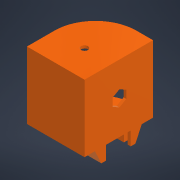
# Autodesk Inventor part: Base
Saved by Autodesk Inventor 2022 (Build 260153000, 153)
## iProperties
Created: 2021-06-04
Part Number: Base
Material: Generic
Document SubType Name: Modeling
Designer: saatvik123
Density: 1 g/cm^3
Appearance: Smooth - Light Orange
Author: saatvik123
## iProperties of the stored document Base_3DPrint.ipt
Created: 2021-06-05
Part Number: Base_3DPrint
Material: Generic
Document SubType Name: Modeling
Designer: sidsa
Density: 1 g/cm^3
Appearance: Default
Author: sidsa
Autodesk Inventor part; units mm, degrees
ref_plane "YZ Plane" through (0, 0, 0) normal (1, 0, 0) x (0, 1, 0)
ref_plane "XZ Plane" through (0, 0, 0) normal (0, 1, 0) x (-1, 0, 0)
ref_plane "XY Plane" through (0, 0, 0) normal (0, 0, 1) x (1, 0, 0)
sketch "Sketch1" plane through (0, 0, 0) normal (0, 0, 1) x (1, 0, 0)
  line L0 (-30.48, 28.575) -> (20.32, 28.575)
  line L1 (20.32, 28.575) -> (20.32, -28.575)
  line L2 (20.32, -28.575) -> (-30.48, -28.575)
  line L3 (-30.48, -28.575) -> (-30.48, 28.575)
  line L4 (-25.4, 28.575) -> (25.4, -28.575) construction
  line L5 (25.4, 28.575) -> (-25.4, -28.575) construction
  line L6 (0, 0) -> (0, -19.5531)
  dimension "d0" = 50.8
  dimension "d1" = 57.15
  dimension "d2" = 20.32
  dimension "d3" = 0
  constraints: 14 end point, 2 midpoint, 2 parallel, 1 horizontal, 1 perpendicular, 1 vertical
  measures "d0" distance of L1.end L2.end
  measures "d1" distance of L0.end L1.end
  measures "d2" distance between parallel lines of L1 L6
  measures "d3" distance of point (0, 0) L6.start
extrude "Extrusion1" add sketch "Sketch1" along normal blind 1.27
sketch "Sketch2" plane through (0, 0, 1.27) normal (0, 0, 1) x (1, 0, 0)
  line L0 (-30.48, -28.575) -> (20.32, -28.575) projected
  line L1 (20.32, -28.575) -> (20.32, 28.575) projected
  line L2 (20.32, 28.575) -> (-30.48, 28.575) projected
  line L3 (-30.48, 28.575) -> (-30.48, -28.575) projected
  line L4 (20.32, 28.575) -> (-30.48, 28.575) projected
  line L5 (-30.48, -28.575) -> (20.32, -28.575) projected
  line L6 (20.32, 28.575) -> (-30.48, 28.575)
  line L7 (-30.48, 28.575) -> (-30.48, -28.575)
  line L8 (-30.48, -28.575) -> (20.32, -28.575)
  line L9 (20.32, -28.575) -> (20.32, 28.575)
  line L10 (22.86, 31.115) -> (-30.48, 31.115)
  line L11 (-30.48, -31.115) -> (22.86, -31.115)
  line L12 (22.86, -31.115) -> (22.86, 31.115)
  line L13 (-30.48, 31.115) -> (-30.48, 28.575)
  line L14 (-30.48, 28.575) -> (-30.48, -28.575) projected
  line L15 (-30.48, -28.575) -> (-30.48, -31.115)
  point P0 (0, 0)
  point P1 (-30.48, 28.575)
  dimension "d6" = 2.54
  dimension "d7" = 2.54
  dimension "d8" = 2.54
  constraints: 18 end point, 3 parallel, 2 horizontal, 2 perpendicular, 1 point on line
  measures "d6" distance between parallel lines of L1 L12
  measures "d7" distance between parallel lines of L2 L10
  measures "d8" distance between parallel lines of L0 L11
extrude "Extrusion2" add sketch "Sketch2" against normal blind 63.5 contours L0 L1 L2 L13 L10 L12 L11 L15
fillet "Fillet1" radius 38.1 2 edges at (-30.48, -29.845, -62.23) (-30.48, 29.845, -62.23)
sketch "Sketch3" plane through (0, 0, 0) normal (0, 0, -1) x (-1, 0, 0)
  line L0 (30.48, -28.575) -> (-20.32, -28.575) projected
  line L1 (30.48, 28.575) -> (30.48, -28.575) projected
  line L2 (-20.32, 28.575) -> (30.48, 28.575) projected
  line L3 (-20.32, -28.575) -> (-20.32, 28.575) projected
  line L4 (-7.62, -31.115) -> (30.48, -31.115) projected
  line L5 (30.48, -31.115) -> (30.48, -28.575) projected
  line L6 (30.48, -28.575) -> (-7.62, -28.575) projected
  line L7 (-7.62, -28.575) -> (-7.62, -31.115) projected
  line L8 (30.48, 31.115) -> (-7.62, 31.115) projected
  line L9 (-7.62, 31.115) -> (-7.62, 28.575) projected
  line L10 (30.48, 28.575) -> (30.48, 28.575) projected
  line L11 (30.48, 28.575) -> (30.48, 31.115) projected
  line L12 (-20.32, 28.575) -> (30.48, 28.575) projected
  line L13 (30.48, 28.575) -> (30.48, 28.575) projected
  line L14 (30.48, -28.575) -> (-20.32, -28.575) projected
  line L15 (26.416, -28.575) -> (23.876, -28.575)
  line L16 (23.876, -28.575) -> (23.876, -26.035)
  line L17 (23.876, -26.035) -> (26.416, -26.035)
  line L18 (26.416, -26.035) -> (26.416, -28.575)
  line L19 (21.336, -28.575) -> (18.796, -28.575)
  line L20 (18.796, -28.575) -> (18.796, -22.225)
  line L21 (18.796, -22.225) -> (21.336, -22.225)
  line L22 (21.336, -22.225) -> (21.336, -28.575)
  line L23 (-20.32, 28.575) -> (30.48, 28.575) projected
  line L24 (26.416, 28.575) -> (23.876, 28.575)
  line L25 (23.876, 28.575) -> (23.876, 26.035)
  line L26 (23.876, 26.035) -> (26.416, 26.035)
  line L27 (26.416, 26.035) -> (26.416, 28.575)
  line L28 (21.336, 28.575) -> (18.796, 28.575)
  line L29 (18.796, 28.575) -> (18.796, 22.225)
  line L30 (18.796, 22.225) -> (21.336, 22.225)
  line L31 (21.336, 22.225) -> (21.336, 28.575)
  point P0 (0, 0)
  point P1 (30.48, -26.035)
  point P2 (23.876, -28.575)
  point P3 (30.48, 26.035)
  point P4 (23.876, 28.575)
  point P5 (21.336, 28.575)
  point P6 (18.796, 28.575)
  dimension "d12" = 2.54
  dimension "d13" = 2.54
  dimension "d14" = 2.54
  dimension "d15" = 6.35
  dimension "d16" = 2.54
  dimension "d17" = 2.54
  dimension "d18" = 2.54
  dimension "d19" = 2.54
  dimension "d20" = 6.35
  dimension "d21" = 2.54
  dimension "d57" = 6.35
  dimension "d58" = 6.35
  dimension "d59" = 4.064
  constraints: 32 end point, 8 parallel, 4 horizontal, 4 perpendicular
  measures "d12" distance of L16.end L17.end
  measures "d13" distance of L15.end L16.end
  measures "d14" distance of L20.end L21.end
  measures "d15" distance of L19.end L20.end
  measures "d16" distance between parallel lines of L16 L22
  measures "d17" distance of L26.end L25.end
  measures "d18" distance of L25.end L24.end
  measures "d19" distance of L30.end L29.end
  measures "d20" distance of L29.end L28.end
  measures "d21" distance between parallel lines of L25 L31
  measures "d57" distance between parallel lines of L21 L0
  measures "d58" distance between parallel lines of L2 L30
  measures "d59" distance between parallel lines of L1 L18
extrude "Extrusion3" add sketch "Sketch3" along normal blind 25.4 contours L0 L16 L17 L18 | L27 L26 L25 L2 | L0 L20 L21 L22 | L31 L30 L29 L2
sketch "Sketch4" plane through (-30.48, -31.115, 1.27) normal (0, -1, 0) x (1, 0, 0)
  arc A0 (35.54, -42.8168) -> (35.14, -42.4168) centre (35.14, -42.8168) ccw
  line L0 (35.54, -42.8168) -> (35.54, -47.1668)
  line L1 (35.54, -47.1668) -> (37.14, -47.1668)
  line L2 (37.14, -47.1668) -> (37.14, -42.8168)
  arc A1 (37.54, -42.4168) -> (37.14, -42.8168) centre (37.54, -42.8168) ccw
  line L3 (37.54, -42.4168) -> (53.14, -42.4168)
  line L4 (53.14, -42.4168) -> (53.14, -20.3168)
  line L5 (53.14, -20.3168) -> (37.54, -20.3168)
  arc A2 (37.14, -19.9168) -> (37.54, -20.3168) centre (37.54, -19.9168) ccw
  line L6 (37.14, -19.9168) -> (37.14, -15.5668)
  line L7 (37.14, -15.5668) -> (35.54, -15.5668)
  line L8 (35.54, -15.5668) -> (35.54, -19.9168)
  arc A3 (35.14, -20.3168) -> (35.54, -19.9168) centre (35.14, -19.9168) ccw
  line L9 (35.14, -20.3168) -> (31.04, -20.3168)
  line L10 (31.04, -20.3168) -> (31.04, -35.0805)
  spline S0 degree 3 poles (31.04, -35.0805) (31.04, -35.2107) (31.032, -35.3398) (31.0199, -35.4684) (31.0078, -35.597) (30.9913, -35.725) (30.9724, -35.8527) (30.9346, -36.1082) (30.8875, -36.3608) (30.84, -36.6168) knots 0 0 0 0 0.249982 0.249982 0.249982 0.499942 0.499942 0.499942 1 1 1 1
  spline S1 degree 3 poles (30.84, -36.6168) (30.8871, -36.8706) (30.9346, -37.1252) (30.9724, -37.3806) (30.9913, -37.5084) (31.0077, -37.6365) (31.0199, -37.7651) (31.032, -37.8937) (31.04, -38.0228) (31.04, -38.153) knots 0 0 0 0 0.5 0.5 0.5 0.750037 0.750037 0.750037 1 1 1 1
  line L11 (31.04, -38.153) -> (31.04, -42.4168)
  line L12 (31.04, -42.4168) -> (35.14, -42.4168)
  line L13 (37.34, -42.8168) -> (37.34, -47.1668)
  line L14 (37.34, -15.5668) -> (37.34, -19.9168)
  line L15 (37.34, -42.8168) -> (53.34, -42.8168)
  line L16 (53.34, -42.8168) -> (53.34, -47.1668)
  line L17 (53.34, -47.1668) -> (37.34, -47.1668)
  line L18 (37.34, -47.1668) -> (37.34, -42.8168)
  line L19 (37.34, -19.9168) -> (53.34, -19.9168)
  line L20 (53.34, -19.9168) -> (53.34, -15.5668)
  line L21 (53.34, -15.5668) -> (37.34, -15.5668)
  line L22 (37.34, -15.5668) -> (37.34, -19.9168)
  line L23 (53.34, 0) -> (53.34, -63.5)
  point P0 (30.48, -1.27)
  dimension "d33" = 0
  dimension "d34" = 0
  constraints: 16 end point, 4 parallel, 2 horizontal, 2 perpendicular
  measures "d33" distance between parallel lines of L23 L16
  measures "d34" distance between parallel lines of L23 L20
extrude "Extrusion4" add sketch "Sketch4" along normal blind 12.7 contours L15 L16 L17 L13 | L21 L20 L19 L14
sketch "Sketch5" plane through (20.32, -28.575, 0) normal (-1, 0, 0) x (0, 0, 1)
  line L0 (0, 0) -> (0, 57.15) projected
  line L1 (0, 57.15) -> (-62.23, 57.15) projected
  line L2 (-62.23, 0) -> (-62.23, 57.15) projected
  line L3 (0, 0) -> (-62.23, 0) projected
  line L4 (-62.23, 59.69) -> (-62.23, -2.54) projected
  line L5 (-62.23, 28.575) -> (-2.2668, 28.575)
  line L6 (-31.1958, 28.575) -> (-31.115, 57.15)
  line L7 (-31.115, 57.15) -> (-37.465, 57.15)
  line L8 (0, 57.15) -> (-62.23, 57.15) projected
  line L9 (-37.465, 57.15) -> (-37.465, 0)
  line L10 (-62.23, 0) -> (-24.13, 0) projected
  line L11 (-37.465, 32.1945) -> (-31.1958, 35.814)
  line L12 (-31.1958, 35.814) -> (-24.9267, 32.1945)
  line L13 (-24.9267, 32.1945) -> (-24.9267, 24.9555)
  line L14 (-24.9267, 24.9555) -> (-31.1958, 21.336)
  line L15 (-31.1958, 21.336) -> (-37.465, 24.9555)
  line L16 (-37.465, 24.9555) -> (-37.465, 32.1945)
  point P0 (0, 28.575)
  point P1 (-37.465, 28.575)
  point P2 (-37.465, 32.1945)
  point P3 (-37.465, 24.9555)
  dimension "d28" = 57.15
  dimension "d30" = 6.35
  dimension "d67" = 7.239
  constraints: 20 end point, 4 midpoint, 3 point on line, 1 coincident, 1 horizontal, 1 perpendicular, 13 other
  measures "d28" distance between parallel lines of L1 L3
  measures "d30" distance of L6.end L7.end
  measures "d67" distance of L15.end L11.start
extrude "Extrusion5" cut sketch "Sketch5" against normal blind 2.54 contours L12 L13 L5 L6 | L6 L5 L9 L11 L12 | L9 L5 L13 L14 L15
sketch "Sketch6" plane through (-30.48, 31.115, 1.27) normal (0, 1, 0) x (1, 0, 0)
  circle A0 centre (29.21, 44.45) radius 2.54
  line L0 (53.34, 0) -> (53.34, 63.5) projected
  line L1 (53.34, 0) -> (0, 0) projected
  point P0 (30.48, 1.27)
  dimension "d38" = 5.08
  dimension "d41" = 24.13
  dimension "d42" = 44.45
  constraints: 1 centre point
  measures "d38" diameter of A0
  measures "d41" distance from line of L0 A0.centre
  measures "d42" distance from line of L1 A0.centre
extrude "Extrusion6" cut sketch "Sketch6" against normal blind 2.54
chamfer "Chamfer3" distance 12.7 angle 25 1 edges at (14.86, -31.115, -45.8968) measured on face at (14.86, -31.615, -45.8968)
chamfer "Chamfer4" distance 12.7 angle 25 1 edges at (14.86, -31.115, -14.2968) measured on face at (14.86, -31.615, -14.2968)
sketch "Sketch8" plane through (-30.48, -43.815, 1.27) normal (0, -1, 0) x (1, 0, 0)
  line L0 (53.34, -42.8168) -> (37.34, -42.8168) projected
  line L1 (50.5178, -53.0889) -> (46.99, -53.0889)
  line L2 (46.99, -53.0889) -> (46.99, -42.8168)
  line L3 (46.99, -42.8168) -> (50.5178, -42.8168)
  line L4 (50.5178, -42.8168) -> (50.5178, -53.0889)
  line L5 (37.34, -53.0889) -> (53.34, -53.0889) projected
  line L6 (53.34, -53.0889) -> (53.34, -47.1668) projected
  point P0 (30.48, -1.27)
  dimension "d52" = 2.8222
  dimension "d53" = 6.35
  constraints: 8 end point, 2 parallel, 1 collinear, 1 horizontal, 1 perpendicular, 1 point on line
  measures "d52" distance between parallel lines of L6 L4
  measures "d53" distance between parallel lines of L6 L2
extrude "Extrusion7" cut sketch "Sketch8" against normal blind 12.7
sketch "Sketch9" plane through (0, 0, 0) normal (0, 0, -1) x (-1, 0, 0)
  line L0 (18.796, -22.225) -> (21.336, -22.225) projected
  line L1 (21.336, -22.225) -> (21.336, -28.575) projected
  line L2 (23.876, -28.575) -> (21.336, -28.575) projected
  line L3 (23.876, -28.575) -> (23.876, -26.035) projected
  line L4 (23.876, -26.035) -> (26.416, -26.035) projected
  line L5 (26.416, -26.035) -> (26.416, -28.575) projected
  line L6 (30.48, -28.575) -> (26.416, -28.575) projected
  line L7 (30.48, 28.575) -> (30.48, -28.575) projected
  line L8 (26.416, 28.575) -> (30.48, 28.575) projected
  line L9 (26.416, 28.575) -> (26.416, 26.035) projected
  line L10 (26.416, 26.035) -> (23.876, 26.035) projected
  line L11 (23.876, 26.035) -> (23.876, 28.575) projected
  line L12 (21.336, 28.575) -> (23.876, 28.575) projected
  line L13 (21.336, 28.575) -> (21.336, 22.225) projected
  line L14 (21.336, 22.225) -> (18.796, 22.225) projected
  line L15 (-20.32, 28.575) -> (18.796, 28.575) projected
  line L16 (-20.32, -28.575) -> (-20.32, 28.575) projected
  line L17 (18.796, -28.575) -> (-20.32, -28.575) projected
  line L18 (18.796, -28.575) -> (18.796, -22.225) projected
  line L19 (18.796, 22.225) -> (18.796, 28.575) projected
  line L20 (-20.32, -28.575) -> (-20.32, 28.575) projected
  line L21 (21.336, -22.225) -> (-20.32, -22.225)
  line L22 (-20.32, -22.225) -> (-20.32, -19.05)
  line L23 (-20.32, -19.05) -> (21.336, -19.05)
  line L24 (21.336, -19.05) -> (21.336, -22.225)
  line L25 (21.336, 22.225) -> (-20.32, 22.225)
  line L26 (-20.32, 22.225) -> (-20.32, 19.05)
  line L27 (-20.32, 19.05) -> (21.336, 19.05)
  line L28 (21.336, 19.05) -> (21.336, 22.225)
  point P0 (0, 0)
  point P1 (-20.32, -22.225)
  dimension "d56" = 6.35
  dimension "d60" = 3.175
  dimension "d61" = 3.175
  constraints: 16 end point, 4 parallel, 2 horizontal, 2 perpendicular, 2 point on line
  measures "d56" distance of L17.start L0.start
  measures "d60" distance of L21.end L22.end
  measures "d61" distance of L26.end L25.end
extrude "Extrusion8" add sketch "Sketch9" along normal blind 25.4 contours L21 L16 L23 L24 L0 | L16 L25 L14 L28 L27
chamfer "Chamfer5" distance 6.35 angle 45 2 edges at (-18.796, -22.225, -12.7) (-18.796, 22.225, -12.7)
sketch "Sketch10" plane through (-30.48, 31.115, 1.27) normal (0, 1, 0) x (1, 0, 0)
  circle A0 centre (29.21, 44.45) radius 2.54 projected
  arc A1 (38.1, 63.5) -> (0, 25.4) centre (38.1, 25.4) ccw projected
  line L0 (0, 0) -> (0, 25.4) projected
  line L1 (53.34, 0) -> (0, 0) projected
  line L2 (53.34, 0) -> (53.34, 63.5) projected
  line L3 (38.1, 63.5) -> (53.34, 63.5) projected
  arc A2 (38.1, 63.5) -> (0, 25.4) centre (38.1, 25.4) ccw projected
  line L4 (26.67, 61.7451) -> (29.21, 59.2051)
  line L5 (26.67, 61.7451) -> (30.2621, 61.7451) construction
  line L6 (29.21, 59.2051) -> (31.75, 62.9671)
  arc A3 (31.75, 62.9671) -> (26.67, 61.7451) centre (38.1, 25.4) ccw
  point P0 (30.48, 1.27)
  dimension "d68" = 45
  constraints: 6 end point, 4 point on circle, 1 centre point, 1 concentric, 1 equal length, 1 horizontal
  measures "d68" angle of L4 L5
extrude "Extrusion9" cut sketch "Sketch10" against normal blind 2.54 contours L6 L4 A1
body "Solid1"
